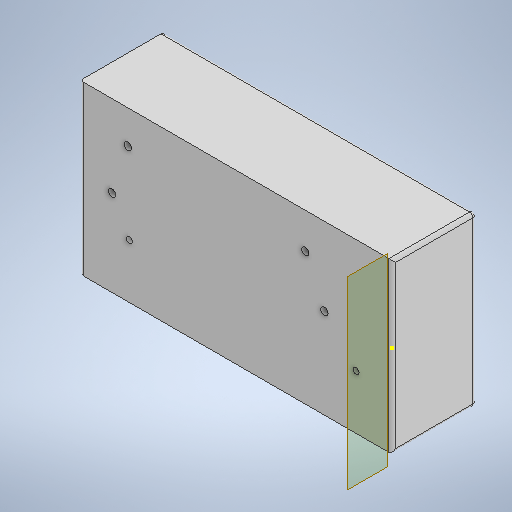
# Autodesk Inventor part: Camera Housing Camera2
Saved by Autodesk Inventor 2025 (Build 290162000, 162)
## iProperties
Created: 2024-07-19
Part Number: Camera Housing Camera2
Material: 일반
Document SubType Name: Modeling
Designer: unney
Density: 1 g/cm^3
Appearance: 기본값
Author: unney
Autodesk Inventor part; units mm, degrees
ref_plane "YZ Plane" through (0, 0, 0) normal (1, 0, 0) x (0, 1, 0)
ref_plane "XZ Plane" through (0, 0, 0) normal (0, 1, 0) x (-1, 0, 0)
ref_plane "XY Plane" through (0, 0, 0) normal (0, 0, 1) x (1, 0, 0)
sketch "스케치1" plane through (0, 0, 0) normal (0, 0, 1) x (1, 0, 0)
  line L0 (-50.4495, 22.5) -> (42.4495, 22.5)
  line L1 (42.4495, 22.5) -> (42.4495, -27.5)
  line L2 (42.4495, -27.5) -> (-50.4495, -27.5)
  line L3 (-50.4495, -27.5) -> (-50.4495, 22.5)
  line L4 (-50.4495, 17.5) -> (37.5505, 17.5)
  line L5 (37.5505, 17.5) -> (37.5505, -22.5)
  line L6 (37.5505, -22.5) -> (-50.4495, -22.5)
  point P0 (0, 0)
  dimension "d0" = 40
  dimension "d1" = 88
  dimension "d2" = 5
  dimension "d3" = 5
  constraints: 14 end point, 4 perpendicular, 2 parallel, 2 point on line, 1 horizontal, 1 vertical
  measures "d0" distance of L4.end L5.end
  measures "d1" distance of L4.start L4.end
  measures "d2" distance between parallel lines of L4 L0
  measures "d3" distance between parallel lines of L2 L6
extrude "돌출1" add sketch "스케치1" against normal blind 6.2 contours L4 L5 L6 L3
extrude "돌출2" add sketch "스케치1" against normal blind 25 contours L0 L1 L2 L3 L6 L5 L4
sketch "스케치2" plane through (0, 0, -6.2) normal (0, 0, -1) x (-1, 0, 0)
  circle A0 centre (36.2565, 12.6083) radius 1.1
  circle A1 centre (-16.5389, 11.9083) radius 1.1
  circle A2 centre (41.0611, -1.7917) radius 1.1
  circle A3 centre (-22.2389, -0.6917) radius 1.1
  circle A4 centre (35.8561, -11.3917) radius 0.9
  circle A5 centre (-31.6439, -11.3917) radius 0.9
  point P0 (0, 0)
  dimension "d8" = 52.8
  dimension "d9" = 2.2
  dimension "d10" = 2.2
  dimension "d11" = 2.2
  dimension "d12" = 2.2
  dimension "d13" = 63.3
  dimension "d14" = 14.4
  dimension "d15" = 12.6
  dimension "d16" = 1.8
  dimension "d17" = 1.8
  dimension "d18" = 67.5
  dimension "d19" = 10.7
  dimension "d23" = 9.405
  dimension "d24" = 0
  dimension "d25" = 0.7
  dimension "d26" = 5.7
  constraints: 6 centre point, 1 other
  measures "d8" distance of A1.centre A0.centre
  measures "d9" diameter of A0
  measures "d10" diameter of A1
  measures "d11" diameter of A2
  measures "d12" diameter of A3
  measures "d13" horizontal distance of A3.centre A2.centre
  measures "d14" vertical distance of A2.centre A0.centre
  measures "d15" vertical distance of A1.centre A3.centre
  measures "d16" diameter of A4
  measures "d17" diameter of A5
  measures "d18" distance of A5.centre A4.centre
  measures "d19" vertical distance of A3.centre A5.centre
  measures "d23" horizontal distance of A3.centre A5.centre
  measures "d24" vertical distance of A5.centre A4.centre
  measures "d25" vertical distance of A1.centre A0.centre
  measures "d26" horizontal distance of A1.centre A3.centre
extrude "돌출3" cut sketch "스케치2" against normal blind 63.3
sketch "스케치3" plane through (42.4495, -27.5, 0) normal (1, 0, 0) x (0, 0, -1)
  line L0 (-14.75, 0) -> (-14.75, 50)
  line L1 (-14.75, 50) -> (39.75, 50)
  line L2 (39.75, 50) -> (39.75, 0)
  line L3 (39.75, 0) -> (-14.75, 0)
  line L4 (0, 0) -> (0, 50) projected
  line L5 (-9.15, 0) -> (-9.15, 50)
  line L6 (34.15, 0) -> (34.15, 50)
  point P0 (0, 27.5)
  dimension "d27" = 54.5
  dimension "d28" = 14.75
  dimension "d29" = 5.6
  dimension "d30" = 43.3
  constraints: 12 end point, 5 perpendicular, 4 point on line, 1 horizontal, 1 vertical
  measures "d27" distance of L0.end L1.end
  measures "d28" distance between parallel lines of L4 L0
  measures "d29" distance between parallel lines of L0 L5
  measures "d30" distance between parallel lines of L6 L5
extrude "돌출4" add sketch "스케치3" along normal blind 10
extrude "돌출5" add sketch "스케치3" along normal blind 80 contours L0 L1 L5 L3 | L6 L1 L2 L3
sketch "스케치4" plane through (42.4495, -27.5, 14.75) normal (0, 0, 1) x (1, 0, 0)
  circle A0 centre (25, 27.5) radius 3.75
  line L0 (0, 50) -> (0, 0) projected
  point P0 (-42.4495, 27.5)
  dimension "d35" = 7.5
  dimension "d36" = 25
  constraints: 1 centre point
  measures "d35" diameter of A0
  measures "d36" distance from line of A0.centre L0
extrude "돌출6" cut sketch "스케치4" against normal blind 80
ref_plane "작업 평면1" through (42.4495, -27.5, 0) normal (-1, 0, 0) x (0, 0, 1)
split "분할1" plane through (42.4495, -27.5, 0) removes the side toward (1, 0, 0)
sketch "스케치5" plane through (42.4495, -27.5, 0) normal (1, 0, 0) x (0, 0, -1)
  point P0 (0, 27.5)
sketch "스케치6" plane through (42.4495, -27.5, 0) normal (1, 0, 0) x (0, 0, -1)
  point P0 (0, 27.5)
fillet "모깎기2" radius 1 15 edges at (-6.4495, -22.5, -25) (37.5505, -2.5, -25) (-6.4495, 17.5, -25) (-4, 22.5, -25) (-50.4495, 20, -25) (-50.4495, -25, -25) (-4, -27.5, -25) (42.4495, -2.5, -25) (42.4495, -2.5, 0) (-50.4495, -2.5, 0) (-50.4495, -2.5, -6.2) (-50.4495, 17.5, -15.6) (-50.4495, -22.5, -15.6) (42.4495, 22.5, -12.5) (42.4495, -27.5, -12.5)
equation "\"d21\" = d13"
